cocked up lcd shit (Autodesk Fusion 360 design; units mm, degrees)
Autodesk Fusion 360 part; units mm, degrees
sketch "Sketch1" plane through (0, 0, 0) normal (0, 1, 0) x (1, 0, 0) in component "Component"
  line L0 (0, 0) -> (60, 0)
  line L1 (60, 0) -> (60, -66)
  line L2 (60, -66) -> (0, -66)
  line L3 (0, -66) -> (0, 0)
  line L4 (0, 0) -> (-2, 0)
  line L5 (0, 0) -> (0, 2)
  line L6 (-2, 2) -> (62, 2)
  line L7 (62, 2) -> (62, -76)
  line L8 (62, -76) -> (-2, -76)
  line L9 (-2, -76) -> (-2, 2)
  line L10 (62, 2) -> (-6, 2)
  line L11 (-6, 2) -> (-6, -76)
  line L12 (-6, -76) -> (62, -76)
  line L13 (62, -76) -> (62, 2)
  line L14 (62, 2) -> (66, 2)
  line L15 (66, 2) -> (66, -76)
  line L16 (66, -76) -> (62, -76)
  line L17 (62, -76) -> (62, 2)
  line L18 (-6, -76) -> (66, -76)
  line L19 (66, -76) -> (66, -77)
  line L20 (66, -77) -> (-6, -77)
  line L21 (-6, -77) -> (-6, -76)
  dimension "d1" = 60
  dimension "d2" = 66
  dimension "d3" = 2
  dimension "d4" = 2
  dimension "d5" = 78
  dimension "d6" = 64
  dimension "d7" = 68
  dimension "d8" = 4
  dimension "d11" = 1
  constraint horizontal L0
  constraint vertical L1
  constraint horizontal L2
  constraint vertical L3
  constraint coincident L0.start L3.end
  constraint horizontal L6
  constraint vertical L7
  constraint horizontal L8
  constraint vertical L9
  constraint horizontal L10
  constraint vertical L11
  constraint horizontal L12
  constraint vertical L13
  constraint horizontal L14
  constraint vertical L15
  constraint horizontal L16
  constraint vertical L17
  constraint horizontal L18
  constraint vertical L19
  constraint horizontal L20
  constraint vertical L21
  measures "d1" distance of L0.start L0.end
  measures "d2" distance of L0.start L2.end
  measures "d3" distance of L0.start L4.end
  measures "d4" distance of L0.start L5.end
  measures "d5" distance of L6.start L8.end
  measures "d6" distance of L6.start L6.end
  measures "d7" distance of L6.end L10.end
  measures "d8" distance of L6.end L14.end
  measures "d11" distance of L11.end L20.end
extrude "Extrude1" add sketch "Sketch1" along normal blind 1.5 contours L4 L5 L6 L7 L8 L9 L10 L12 L13 L17 L18 | L4 L5 L6 L9 L10 | L9 L10 L11 L12 L18 | L7 L13 L14 L15 L16 L17 L18 in component "Component"
extrude "Extrude2" add sketch "Sketch1" along normal blind 1.5 contours L8 L12 L16 L18 L19 L20 L21 in component "Component"
component "Component" placed x (1, 0, 0) y (0, 1, 0) z (0, 0, 1) at (0, 0, 0)
equation "d5 = 66 mm + 12 mm"
